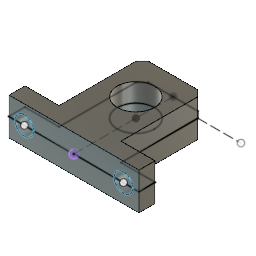
Soporte de Varilla v4 (Autodesk Fusion 360 design; units mm, degrees)
Autodesk Fusion 360 part; units mm, degrees
sketch "Boceto1" plane through (0, 0, 0) normal (0, 0, 1) x (1, 0, 0)
  line L0 (0, 0) -> (21, 0)
  line L1 (21, 0) -> (21, 5.2)
  line L2 (21, 5.2) -> (10, 5.2)
  line L3 (10, 5.2) -> (10, 30)
  line L4 (10, 30) -> (8, 32)
  line L5 (10, 30) -> (23.9079, 30) construction
  line L6 (8, 32) -> (0, 32)
  line L7 (0, 0) -> (0, 32) construction
  line L8 (-10, 30) -> (-8, 32)
  line L9 (-10, 5.2) -> (-10, 30)
  line L10 (-21, 0) -> (-21, 5.2)
  line L11 (-21, 5.2) -> (-10, 5.2)
  line L12 (-8, 32) -> (0, 32)
  circle A0 centre (0, 20) radius 6
  line L13 (0, 0) -> (-21, 0)
  dimension "d17" = 5.2
  dimension "d19" = 45
  dimension "d20" = 8
  dimension "d21" = 32
  dimension "d24" = 10
  dimension "d25" = 12
  dimension "d26" = 20
  dimension "d47" = 10
  dimension "d50" = 11
  constraint coincident L0.start L7.start
  constraint horizontal L0
  constraint perpendicular L0 L1
  constraint perpendicular L1 L2
  constraint perpendicular L2 L3
  constraint horizontal L5
  constraint perpendicular L3 L6
  constraint symmetric L0.end L7 L10.start
  constraint symmetric L1.end L7 L10.end
  constraint symmetric L2.end L7 L9.start
  constraint symmetric L3.end L7 L8.start
  constraint symmetric L4.end L7 L8.end
  constraint symmetric L6.end L7 L12.end
  constraint coincident L7 A0.centre
  measures "d17" distance of L0.end L1.end
  measures "d19" angle of L4 L5
  measures "d20" distance of L4.end L6.end
  measures "d21" distance of L0 L6
  measures "d24" distance of L3.end L7
  measures "d25" diameter of A0
  measures "d26" distance of L0.start A0.centre
  measures "d47" distance of L0.start L3
  measures "d50" distance of L9 L10
extrude "Extruir2" add sketch "Boceto1" along normal mid plane 12
sketch "Boceto7" plane through (0, 0, 0) normal (0, -1, 0) x (1, 0, 0)
  line L0 (21, -6) -> (21, 6)
  line L1 (21, 6) -> (-21, 6)
  line L2 (-21, 6) -> (-21, -6)
  line L3 (-21, -6) -> (21, -6)
  circle A0 centre (16, 0) radius 3
  circle A1 centre (-16, 0) radius 3
  dimension "d57" = 6
  dimension "d58" = 5
  dimension "d59" = 6
  measures "d57" diameter of A0
  measures "d58" distance of L0 A0.centre
  measures "d59" diameter of A1
extrude "Extruir11" cut sketch "Boceto7" along normal mid plane 52 contours A0 | A1
extrude "Extruir6" [suppressed]
extrude "Extruir7" [suppressed]
component "Component" placed x (1, 0, 0) y (0, 1, 0) z (0, 0, 1) at (0, 0, 0)
